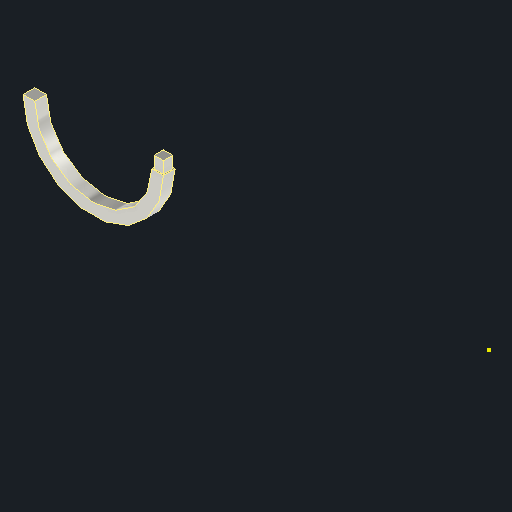
# Autodesk Inventor part: McCrea_kabel_walle
Saved by Autodesk Inventor 2022 (Build 260153000, 153)
## iProperties
Created: 2022-01-17
Part Number: McCrea_kabel_walle
Material: Generic
Document SubType Name: Modeling
Designer: student
Density: 1 g/cm^3
Appearance: Silver
Author: student
Autodesk Inventor part; units mm, degrees
ref_plane "YZ Plane" through (0, 0, 0) normal (1, 0, 0) x (0, 1, 0)
ref_plane "XZ Plane" through (0, 0, 0) normal (0, 1, 0) x (-1, 0, 0)
ref_plane "XY Plane" through (0, 0, 0) normal (0, 0, 1) x (1, 0, 0)
sketch "Sketch1" plane through (0, 0, 0) normal (0, 0, 1) x (1, 0, 0)
  arc A0 (-38.8309, 24) -> (-26.8309, 24) centre (-32.8309, 24) ccw
  arc A1 (-37.8309, 24) -> (-27.8309, 24) centre (-32.8309, 24) ccw
  line L0 (-38.8309, 24) -> (-26.8309, 24)
  point P0 (0, 0)
  dimension "d0" = 1
  dimension "d1" = 5
  constraints: 4 point on circle, 2 centre point, 2 end point, 2 point on line, 1 coincident, 1 horizontal
  measures "d0" radial gap between concentric circles of A0 A1
  measures "d1" radius of A1
ref_plane "Work Plane1" through (-32.8309, 24, 0) normal (0, 1, 0) x (-1, 0, 0)
sketch "Sketch2" plane through (-32.8309, 24, 0) normal (0, 1, 0) x (-1, 0, 0)
  point P0 (-32.8309, 0)
extrude "Extrusion1" add sketch "Sketch1" along normal blind 1 contours L0 A1 A0
sketch "Sketch3" plane through (-27.8309, 24, 0) normal (0, 1, 0) x (1, 0, 0)
  line L0 (1, 0) -> (0, 0) projected
  line L1 (0, 0) -> (0, -1) projected
  line L2 (1, -1) -> (0, -1) projected
  line L3 (1, 0) -> (1, -1) projected
  line L4 (0.1, -0.1) -> (0.9, -0.1)
  line L5 (0.9, -0.1) -> (0.9, -0.9)
  line L6 (0.9, -0.9) -> (0.1, -0.9)
  line L7 (0.1, -0.9) -> (0.1, -0.1)
  point P0 (27.8309, 0)
  dimension "d4" = 0.8
  constraints: 8 end point, 3 other
  measures "d4" distance of L4.start L4.end
extrude "Extrusion2" add sketch "Sketch3" along normal blind 1 contours L4 L5 L6 L7
body "Solid1"
